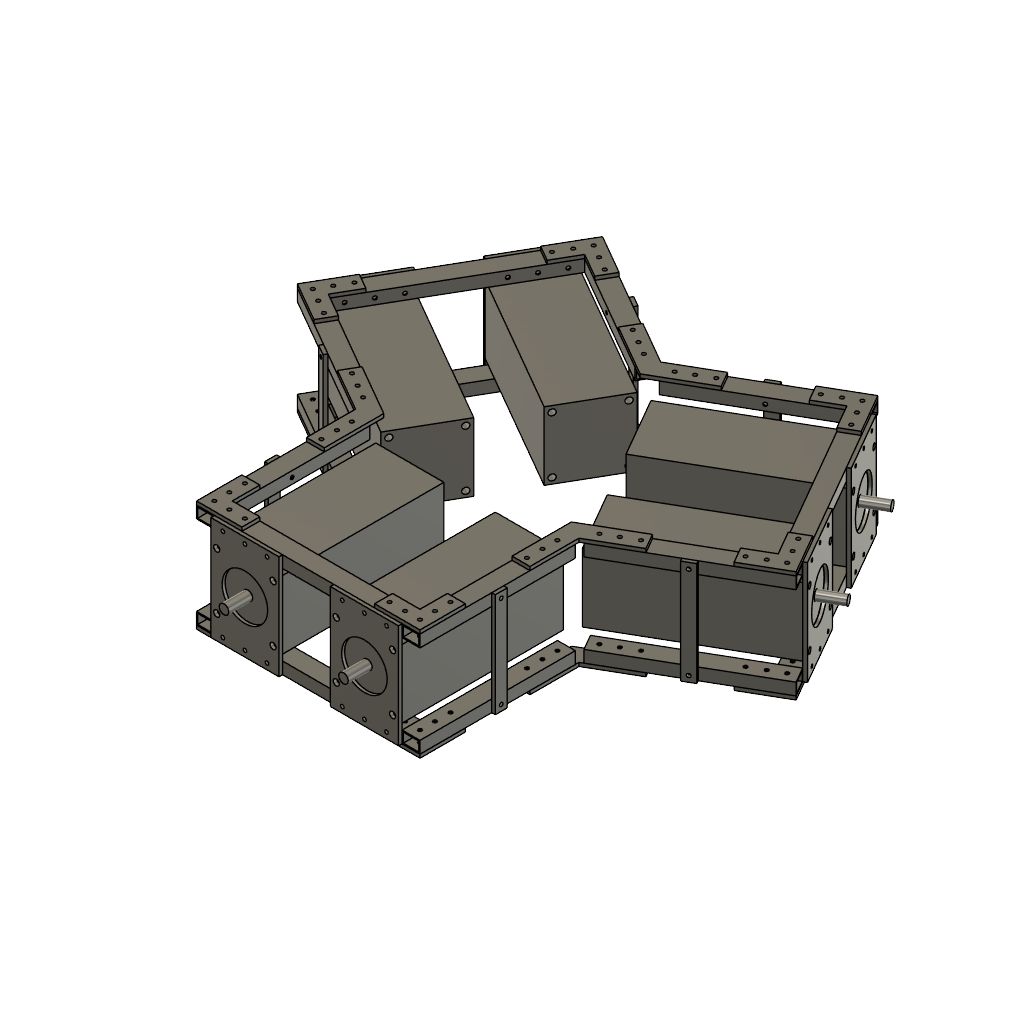
Base (Autodesk Fusion 360 design; units mm, degrees)
Autodesk Fusion 360 part; units mm, degrees
note: some values were not read from the file. Chosen so that the rebuilt part matches the saved one: which bodies a step acts on. Set by a fixed rule: which sketch regions a step uses.
sketch "Sketch1" plane through (0, 0, 0) normal (0, 1, 0) x (1, 0, 0)
  line L0 (0, 0) -> (0, -200)
  line L1 (-50, -200) -> (55.0397, -200)
  line L2 (-21.5, -187) -> (-78.5, -187)
  line L3 (-78.5, -187) -> (-78.5, -52)
  line L4 (-21.5, -187) -> (-21.5, -52)
  line L5 (-78.5, -52) -> (-21.5, -52)
  constraint coincident L0.start origin
  constraint vertical L0
  constraint perpendicular L0 L1
  constraint parallel L1 L2
  constraint perpendicular L2 L3
  constraint perpendicular L2 L4
extrude "Extrude1" add sketch "Sketch1" along normal blind 28.5 makes body 1
move_face "OffsetFaces1" offset 28.5 1 faces at (-59.5, 0, 97) on bodies 1
sketch "Sketch2" plane through (0, 0, 187) normal (0, 0, 1) x (1, 0, 0)
  line L0 (-78.5, -28.5) -> (-21.5, -28.5)
  line L1 (-21.5, -28.5) -> (-21.5, 28.5)
  line L2 (-21.5, 28.5) -> (-78.5, 28.5)
  line L3 (-78.5, 28.5) -> (-78.5, -28.5)
  line L4 (-78.5, 28.5) -> (-21.5, -28.5)
  line L5 (-21.5, 28.5) -> (-78.5, -28.5)
  circle A0 centre (-50, 0) radius 19.05
  constraint coincident L2.end L3.start
  constraint coincident L0.end L1.start
  constraint coincident L1.end L2.start
  constraint coincident L0.start L3.end
  constraint midpoint L5 A0.centre
extrude "Extrude2" add sketch "Sketch2" along normal blind 0.5 contours L4 L5 A0 | L4 L5 A0 | L4 L5 A0 | L4 L5 A0 bodies 1
sketch "Sketch3" plane through (0, 0, 187) normal (0, 0, 1) x (1, 0, 0)
  circle A0 centre (-50, 0) radius 19.05
  line L0 (-78.5, -28.5) -> (-21.5, -28.5)
  line L1 (-21.5, -28.5) -> (-21.5, 28.5)
  line L2 (-21.5, 28.5) -> (-78.5, 28.5)
  line L3 (-78.5, 28.5) -> (-78.5, -28.5)
  line L4 (-26.43, 23.57) -> (-26.43, -23.57)
  line L5 (-26.43, -23.57) -> (-73.57, -23.57)
  line L6 (-73.57, -23.57) -> (-73.57, 23.57)
  line L7 (-73.57, 23.57) -> (-26.43, 23.57)
  circle A1 centre (-73.57, 23.57) radius 2.55
  circle A2 centre (-26.43, 23.57) radius 2.55
  circle A3 centre (-26.43, -23.57) radius 2.55
  circle A4 centre (-73.57, -23.57) radius 2.55
  constraint perpendicular L2 L4
  constraint perpendicular L4 L5
  constraint perpendicular L5 L6
  constraint perpendicular L4 L7
  constraint coincident L6.end L7.start
  constraint coincident L4.start L7.end
  constraint coincident L4.end L5.start
  constraint coincident L5.end L6.start
extrude "Extrude3" cut sketch "Sketch3" against normal blind 135 contours L4 L7 A2 | L4 L7 A2 | L4 L5 A3 | L4 L5 A3 | L6 L7 A1 | L6 L7 A1 | L5 L6 A4 | L5 L6 A4 bodies 1
sketch "Sketch4" plane through (0, 0, 187.5) normal (0, 0, 1) x (1, 0, 0)
  circle A0 centre (-50, 0) radius 19.05
  circle A1 centre (-50, 0) radius 4
  constraint concentric A0 A1
extrude "Extrude4" add sketch "Sketch4" along normal blind 20 contours A1 bodies 1
mirror "Mirror1" about plane through (0, 0, 0) normal (1, 0, 0) of bodies 1 makes body 2
pattern_circular "C-Pattern1" count 3 over 360 about axis through (0, 1.75, 0) along (0, 1, 0) of bodies 1 2 makes body 3 at (113.7545, 28.5, 3.0285) makes body 4 at (-102.7256, 28.5, -106.074) makes body 5 at (54.2545, 28.5, -100.0285) makes body 6 at (-113.7545, 28.5, 3.0285)
sketch "Sketch5" plane through (0, 0, 187) normal (0, 0, 1) x (1, 0, 0)
  circle A0 centre (-73.57, 23.57) radius 2.55
  circle A1 centre (-26.43, 23.57) radius 2.55
  circle A2 centre (-73.57, -23.57) radius 2.55
  circle A3 centre (-26.43, -23.57) radius 2.55
  circle A4 centre (-50, 0) radius 19.05
  line L0 (-78.5, -28.5) -> (-21.5, -28.5)
  line L1 (-21.5, -28.5) -> (-21.5, 28.5)
  line L2 (-21.5, 28.5) -> (-78.5, 28.5)
  line L3 (-78.5, 28.5) -> (-78.5, -28.5)
  line L4 (-83.4322, 43.5) -> (-5, 43.5)
  line L5 (-81, -43.5) -> (-19, -43.5)
  line L6 (-78.5, -28.5) -> (-78.5, -50)
  line L7 (-21.5, -28.5) -> (-21.5, -50)
  line L8 (-21.5, 28.5) -> (-21.5, 50)
  line L9 (-78.5, 28.5) -> (-78.5, 53)
  constraint horizontal L4
  constraint horizontal L5
  constraint coincident L0.start L3.end
  constraint perpendicular L0 L6
  constraint coincident L0.end L1.start
  constraint perpendicular L0 L7
  constraint coincident L1.end L2.start
  constraint perpendicular L2 L8
  constraint coincident L2.end L3.start
  constraint perpendicular L4 L9
extrude "Extrude5" add sketch "Sketch5" along normal blind 3 separate body makes body 7
sketch "Sketch6" plane through (0, 0, 190) normal (0, 0, 1) x (1, 0, 0)
  circle A0 centre (-73.57, 23.57) radius 2.55
  circle A1 centre (-26.43, 23.57) radius 2.55
  circle A2 centre (-26.43, -23.57) radius 2.55
  circle A3 centre (-73.57, -23.57) radius 2.55
  circle A4 centre (-50, 0) radius 19.05
  line L0 (-78.5, 43.5) -> (-78.5, -43.5)
  line L1 (-78.5, -43.5) -> (-21.5, -43.5)
  line L2 (-21.5, -43.5) -> (-21.5, 43.5)
  line L3 (-21.5, 43.5) -> (-78.5, 43.5)
  line L4 (-82, 38.5) -> (-14, 38.5)
  circle A5 centre (-68.5, 38.5) radius 1.5
  circle A6 centre (-31.5, 38.5) radius 1.5
  circle A7 centre (-50, 38.5) radius 1.5
  line L5 (-82.4543, -38.5) -> (-13.292, -38.5) construction
  line L6 (-50, 38.5) -> (-50, -43) construction
  line L7 (-31.5, 38.5) -> (-31.5, -43) construction
  line L8 (-68.5, 38.5) -> (-68.5, -42) construction
  circle A8 centre (-68.5, -38.5) radius 1.5
  circle A9 centre (-50, -38.5) radius 1.5
  circle A10 centre (-31.5, -38.5) radius 1.5
  constraint horizontal L4
  constraint coincident L4 A5.centre
  constraint coincident L4 A6.centre
  constraint coincident L4 A7.centre
  constraint perpendicular L0 L5
  constraint coincident A7.centre L6.start
  constraint perpendicular L1 L6
  constraint coincident A6.centre L7.start
  constraint perpendicular L5 L7
  constraint coincident A5.centre L8.start
  constraint perpendicular L1 L8
  constraint coincident L8 A8.centre
  constraint coincident L5 A8.centre
  constraint coincident L6 A9.centre
  constraint coincident L5 A9.centre
  constraint coincident L7 A10.centre
  constraint coincident L5 A10.centre
extrude "Extrude6" cut sketch "Sketch6" against normal blind 3 contours L4 A5 | L4 A5 | L4 A6 | L4 A6 | L4 A7 | L4 A7 | A8 | A9 | A10 bodies 7
sketch "Sketch7" plane through (0, 0, 187) normal (0, 0, -1) x (-1, 0, 0)
  circle A0 centre (31.5, -38.5) radius 1.5
  circle A1 centre (68.5, 38.5) radius 1.5
  circle A2 centre (50, -38.5) radius 1.5
  circle A3 centre (31.5, 38.5) radius 1.5
  circle A4 centre (50, 38.5) radius 1.5
  circle A5 centre (68.5, -38.5) radius 1.5
  circle A6 centre (73.57, 23.57) radius 2.55
  circle A7 centre (26.43, 23.57) radius 2.55
  circle A8 centre (26.43, -23.57) radius 2.55
  circle A9 centre (73.57, -23.57) radius 2.55
  circle A10 centre (50, 0) radius 19.05
  line L0 (78.5, -43.5) -> (78.5, 43.5)
  line L1 (78.5, 43.5) -> (21.5, 43.5)
  line L2 (21.5, 43.5) -> (21.5, -43.5)
  line L3 (21.5, -43.5) -> (78.5, -43.5)
  line L4 (21.5, 43.5) -> (78.5, 43.5)
  line L5 (78.5, 43.5) -> (78.5, 28.5)
  line L6 (78.5, 28.5) -> (21.5, 28.5)
  line L7 (21.5, 28.5) -> (21.5, 43.5)
  line L8 (18.6686, 33.5) -> (82.3438, 33.5)
  line L9 (-78.5, -28.5) -> (-78.5, 28.5)
  line L10 (-78.5, -7.8499) -> (-78.5, 65.8048)
  line L11 (18.6686, 33.5) -> (-88, 33.5)
  line L12 (21.5, 43.5) -> (-81.618, 43.5)
  constraint horizontal L4
  constraint vertical L5
  constraint horizontal L6
  constraint vertical L7
  constraint coincident L0 L5.end
  constraint coincident L1.end L2.start
  constraint perpendicular L2 L8
  constraint coincident L9 L10.start
  constraint perpendicular L2 L11
  constraint perpendicular L2 L12
extrude "Extrude7" add sketch "Sketch7" along normal blind 15 separate body contours L0 L1 L2 L4 L5 L7 L8 makes body 8
sketch "Sketch8" plane through (-78.5, 0, 0) normal (-1, 0, 0) x (0, 0, 1)
  line L0 (187, 33.5) -> (187, 43.5)
  line L1 (187, 43.5) -> (172, 43.5)
  line L2 (172, 43.5) -> (172, 33.5)
  line L3 (172, 33.5) -> (187, 33.5)
mirror "Mirror2" about plane through (0, 0, 0) normal (1, 0, 0) of bodies 7 makes body 9
pattern_circular "C-Pattern2" count 3 over 360 about axis through (0, 1.75, 0) along (0, 1, 0) of bodies 9 7 makes body 10 at (191.19, 30.8975, -42.8491) makes body 11 at (-132.7035, 30.8975, -144.1509) makes body 12 at (132.7035, -30.8975, -144.1509) makes body 13 at (-191.19, 30.8975, -42.8491)
sketch "Sketch9" plane through (-21.5, 0, 0) normal (1, 0, 0) x (0, 0, -1)
  line L0 (-187, 43.5) -> (-187, 33.5)
  line L1 (-187, 33.5) -> (-172, 33.5)
  line L2 (-172, 33.5) -> (-172, 43.5)
  line L3 (-172, 43.5) -> (-187, 43.5)
sketch "Sketch10" plane through (-21.5, 0, 0) normal (1, 0, 0) x (0, 0, -1)
  line L0 (-187, 43.5) -> (-187, 33.5)
  line L1 (-187, 33.5) -> (-172, 33.5)
  line L2 (-172, 33.5) -> (-172, 43.5)
  line L3 (-172, 43.5) -> (-187, 43.5)
extrude "Extrude8" add sketch "Sketch10" along normal blind 100 separate body makes body 14
combine "Combine1" operation add target body 14 tool bodies 8
sketch "Sketch11" plane through (0, 0, 172) normal (0, 0, -1) x (-1, 0, 0)
  circle A0 centre (31.5, 38.5) radius 1.5
  circle A1 centre (68.5, 38.5) radius 1.5
  circle A2 centre (50, 38.5) radius 1.5
  line L0 (78.5, 43.5) -> (-78.5, 43.5)
  line L1 (-78.5, 43.5) -> (-78.5, 33.5)
  line L2 (-78.5, 33.5) -> (78.5, 33.5)
  line L3 (78.5, 33.5) -> (78.5, 43.5)
  circle A3 centre (-68.5, 38.5) radius 1.5
  circle A4 centre (-50, 38.5) radius 1.5
  circle A5 centre (-31.5, 38.5) radius 1.5
extrude "Extrude9" cut sketch "Sketch11" against normal blind 15 contours A3 | A4 | A5 bodies 14
sketch "Sketch12" plane through (78.5, 0, 0) normal (1, 0, 0) x (0, 0, -1)
  line L0 (-172, 43.5) -> (-187, 43.5)
  line L1 (-187, 43.5) -> (-187, 33.5)
  line L2 (-187, 33.5) -> (-172, 33.5)
  line L3 (-172, 33.5) -> (-172, 43.5)
  line L4 (-187, 43.5) -> (-172, 33.5) construction
  line L5 (-172, 43.5) -> (-187, 33.5) construction
  line L6 (-173, 34.6971) -> (-186, 34.6971)
  line L7 (-186, 34.6971) -> (-186, 42.3029)
  line L8 (-186, 42.3029) -> (-173, 42.3029)
  line L9 (-173, 42.3029) -> (-173, 34.6971)
  line L10 (-173, 34.6971) -> (-186, 42.3029) construction
  line L11 (-186, 34.6971) -> (-173, 42.3029) construction
  point P0 (-179.5, 38.5)
  constraint coincident L0.end L1.start
  constraint coincident L2.end L3.start
  constraint coincident L0.start L3.end
  constraint coincident L1.end L2.start
  constraint horizontal L6
  constraint perpendicular L6 L7
  constraint parallel L6 L8
  constraint parallel L7 L9
  constraint coincident L10 P0
  constraint coincident L11 P0
  constraint midpoint L4 P0
extrude "Extrude10" cut sketch "Sketch12" against normal blind 157 contours L6 L7 L8 L9 bodies 14
sketch "Sketch13" plane through (0, 43.5, 0) normal (0, 1, 0) x (-1, 0, 0)
  line L0 (78.5, 187) -> (-78.5, 187)
  line L1 (-78.5, 187) -> (-78.5, 172)
  line L2 (-78.5, 172) -> (78.5, 172)
  line L3 (78.5, 172) -> (78.5, 187)
  line L4 (55.5, 187) -> (55.5, 172)
  line L5 (73.5, 172) -> (73.5, 187)
  line L6 (60.5, 172) -> (60.5, 187)
  line L7 (78.5, 179.5) -> (42, 179.5) construction
  circle A0 centre (60.5, 179.5) radius 1.5
  circle A1 centre (73.5, 179.5) radius 1.5
  line L8 (-73.5, 170) -> (-73.5, 191.2078)
  line L9 (-60.5, 169.8695) -> (-60.5, 193.8538)
  line L10 (-55.5, 170) -> (-55.5, 195.9898)
  line L11 (-78.5, 179.5) -> (-48.9118, 179.5) construction
  circle A2 centre (-73.5, 179.5) radius 1.5
  circle A3 centre (-60.5, 179.5) radius 1.5
  constraint coincident L0 L4.start
  constraint coincident L2 L4.end
  constraint perpendicular L2 L4
  constraint coincident L2 L5.start
  constraint coincident L0 L5.end
  constraint perpendicular L0 L5
  constraint coincident L2 L6.start
  constraint coincident L0 L6.end
  constraint perpendicular L0 L6
  constraint midpoint L3 L7.start
  constraint perpendicular L3 L7
  constraint midpoint L6 A0.centre
  constraint midpoint L5 A1.centre
  constraint perpendicular L2 L8
  constraint perpendicular L2 L9
  constraint perpendicular L0 L10
  constraint midpoint L1 L11.start
  constraint perpendicular L10 L11
  constraint coincident L8 A2.centre
  constraint coincident L11 A2.centre
  constraint coincident L9 A3.centre
  constraint coincident L11 A3.centre
extrude "Extrude11" cut sketch "Sketch13" against normal blind 10 contours L5 A1 | L5 A1 | L6 A0 | L6 A0 | L9 A3 | L9 A3 | L8 A2 | L8 A2 bodies 14
pattern_circular "C-Pattern3" count 3 over 360 about axis through (0, 1.75, 0) along (0, 1, 0) of bodies 14 makes body 15 at (170.2315, 33.5, -75.1252) makes body 16 at (-150.1761, 33.5, -109.8622)
mirror "Mirror3" about plane through (0, 0, 0) normal (0, 1, 0) of bodies 14 16 15 makes body 17 at (-20.0122, -33.5, 174.0245) makes body 18 at (170.2315, -33.5, -75.1252) makes body 19 at (-150.1761, -33.5, -109.8622)
sketch "Sketch14" plane through (0, 43.5, 0) normal (0, 1, 0) x (-1, 0, 0)
  circle A0 centre (-73.5, 179.5) radius 1.5
  circle A1 centre (73.5, 179.5) radius 1.5
  circle A2 centre (-60.5, 179.5) radius 1.5
  circle A3 centre (60.5, 179.5) radius 1.5
  line L0 (78.5, 187) -> (-78.5, 187)
  line L1 (-78.5, 187) -> (-78.5, 172)
  line L2 (-78.5, 172) -> (78.5, 172)
  line L3 (78.5, 172) -> (78.5, 187)
  line L4 (55.5, 187) -> (55.5, 172)
  circle A4 centre (60.5, 179.5) radius 1.5
  circle A5 centre (73.5, 179.5) radius 1.5
  line L5 (55.5, 187) -> (93.5, 187)
  line L6 (93.5, 187) -> (93.5, 149)
  line L7 (93.5, 149) -> (78.5, 149)
  line L8 (78.5, 149) -> (78.5, 172)
  line L9 (60.5, 179.5) -> (97, 179.5) construction
  line L10 (96, 154) -> (76, 154) construction
  line L11 (97, 167) -> (74, 167) construction
  line L12 (86, 149) -> (86, 187) construction
  circle A6 centre (86, 179.5) radius 1.5
  circle A7 centre (86, 167) radius 1.5
  circle A8 centre (86, 154) radius 1.5
  constraint coincident L4.start L5.start
  constraint perpendicular L3 L5
  constraint vertical L6
  constraint perpendicular L6 L7
  constraint coincident L2.end L3.start
  constraint coincident A3.centre A4.centre
  constraint perpendicular L6 L9
  constraint perpendicular L6 L10
  constraint perpendicular L8 L11
  constraint midpoint L7 L12.start
  constraint coincident L5 L12.end
  constraint perpendicular L5 L12
  constraint coincident L12 A6.centre
  constraint coincident L9 A6.centre
  constraint coincident L12 A7.centre
  constraint coincident L11 A7.centre
  constraint midpoint L10 A8.centre
extrude "Extrude12" add sketch "Sketch14" along normal blind 3 separate body contours L0 L2 L3 L4 L5 | L3 L5 L6 L7 L8 makes body 20
sketch "Sketch15" plane through (0, 43.5, 0) normal (0, -1, 0) x (1, 0, 0)
  circle A0 centre (-86, 179.5) radius 1.5
  circle A1 centre (-86, 154) radius 1.5
  circle A2 centre (-86, 167) radius 1.5
  circle A3 centre (-60.5, 179.5) radius 1.5
  circle A4 centre (-73.5, 179.5) radius 1.5
  line L0 (-55.5, 172) -> (-55.5, 187)
  line L1 (-55.5, 187) -> (-93.5, 187)
  line L2 (-93.5, 187) -> (-93.5, 149)
  line L3 (-93.5, 149) -> (-78.5, 149)
  line L4 (-78.5, 149) -> (-78.5, 172)
  line L5 (-78.5, 172) -> (-55.5, 172)
  line L6 (-21.5, 52) -> (-21.5, 187)
  line L7 (-21.5, 187) -> (-78.5, 187)
  line L8 (-78.5, 187) -> (-78.5, 52)
  line L9 (-78.5, 52) -> (-21.5, 52)
  line L10 (-93.5, 187) -> (-78.5, 187)
  line L11 (-78.5, 187) -> (-78.5, 52)
  line L12 (-78.5, 52) -> (-93.5, 52)
  line L13 (-93.5, 52) -> (-93.5, 187)
  line L14 (-96, 57) -> (-76, 57)
  constraint horizontal L10
  constraint vertical L11
  constraint horizontal L12
  constraint vertical L13
  constraint coincident L8.end L9.start
  constraint coincident L1.end L2.start
  constraint perpendicular L11 L14
extrude "Extrude13" add sketch "Sketch15" along normal blind 10 separate body contours L1 L2 L3 L4 L8 L10 L11 L13 | L3 L8 L11 L13 L14 makes body 21
sketch "Sketch16" plane through (0, 43.5, 0) normal (0, 1, 0) x (-1, 0, 0)
  circle A0 centre (86, 154) radius 1.5
  circle A1 centre (86, 167) radius 1.5
  circle A2 centre (86, 179.5) radius 1.5
  line L0 (93.5, 57) -> (93.5, 187)
  line L1 (93.5, 187) -> (78.5, 187)
  line L2 (78.5, 187) -> (78.5, 57)
  line L3 (78.5, 122) -> (93.5, 122)
  circle A3 centre (86, 90) radius 1.5
  circle A4 centre (86, 77) radius 1.5
  circle A5 centre (86, 64.5) radius 1.5
  line L4 (78.5, 57) -> (93.5, 57)
  constraint midpoint L2 L3.start
  constraint midpoint L0 L3.end
  constraint symmetric A0 L3 A3
  constraint symmetric A1 L3 A4
  constraint symmetric A2 L3 A5
extrude "Extrude14" cut sketch "Sketch16" against normal blind 10 contours A3 | A4 | A5 bodies 21
sketch "Sketch17" plane through (0, 0, 187) normal (0, 0, 1) x (1, 0, 0)
  line L0 (-78.5, 43.5) -> (-93.5, 43.5)
  line L1 (-93.5, 43.5) -> (-93.5, 33.5)
  line L2 (-93.5, 33.5) -> (-78.5, 33.5)
  line L3 (-78.5, 33.5) -> (-78.5, 43.5)
  line L4 (-93.5, 43.5) -> (-78.5, 33.5) construction
  line L5 (-93.5, 33.5) -> (-78.5, 43.5) construction
  line L6 (-79.5, 34.5) -> (-92.5, 34.5)
  line L7 (-92.5, 34.5) -> (-92.5, 42.5)
  line L8 (-92.5, 42.5) -> (-79.5, 42.5)
  line L9 (-79.5, 42.5) -> (-79.5, 34.5)
  line L10 (-79.5, 34.5) -> (-92.5, 42.5) construction
  line L11 (-92.5, 34.5) -> (-79.5, 42.5) construction
  point P0 (-86, 38.5)
  constraint coincident L0.end L1.start
  constraint coincident L2.end L3.start
  constraint coincident L1.end L2.start
  constraint coincident L0.start L3.end
  constraint horizontal L6
  constraint perpendicular L6 L7
  constraint parallel L6 L8
  constraint parallel L7 L9
  constraint coincident L10 P0
  constraint coincident L11 P0
  constraint midpoint L4 P0
extrude "Extrude15" cut sketch "Sketch17" against normal blind 135 contours L6 L7 L8 L9 bodies 21
mirror "Mirror4" about plane through (0, 0, 0) normal (1, 0, 0) of bodies 21 20 makes body 22 at (91.5, 46.5, 167.6667) makes body 23 at (83.7518, 43.5, 131.0107)
mirror "Mirror5" about plane through (0, 0, 0) normal (0, 1, 0) of bodies 21 20 22 23 makes body 24 at (-91.5, -46.5, 167.6667) makes body 25 at (-83.7518, -43.5, 131.0107) makes body 26 at (91.5, -46.5, 167.6667) makes body 27 at (83.7518, -43.5, 131.0107)
pattern_circular "C-Pattern4" count 3 over 360 about axis through (0, 1.75, 0) along (0, 1, 0) of bodies 21 20 22 23 27 25 24 26 makes body 28 at (190.9536, 46.5, -4.592) makes body 29 at (-99.4536, 46.5, -163.0747) makes body 30 at (155.3516, 43.5, 7.0501) makes body 31 at (-71.5702, 33.5, -138.0635) makes body 32 at (99.4536, 46.5, -163.0747) makes body 33 at (-190.9536, 46.5, -4.592) makes body 34 at (71.5702, 43.5, -138.0635) makes body 35 at (-155.3516, 43.5, 7.0501) makes body 36 at (190.9536, -46.5, -4.592) makes body 37 at (-99.4536, -46.5, -163.0747) makes body 38 at (155.3516, -43.5, 7.0501) makes body 39 at (-71.5702, -33.5, -138.0635) makes body 40 at (99.4536, -46.5, -163.0747) makes body 41 at (-190.9536, -46.5, -4.592) makes body 42 at (71.5702, -43.5, -138.0635) makes body 43 at (-155.3516, -43.5, 7.0501)
sketch "Sketch18" plane through (0, 43.5, 0) normal (0, 1, 0) x (-1, 0, 0)
  circle A0 centre (86, 64.5) radius 1.5
  circle A1 centre (86, 77) radius 1.5
  circle A2 centre (86, 90) radius 1.5
  circle A3 centre (86, 167) radius 1.5
  circle A4 centre (86, 179.5) radius 1.5
  circle A5 centre (86, 154) radius 1.5
  line L0 (78.5, 57) -> (93.5, 57)
  line L1 (93.5, 57) -> (93.5, 187)
  line L2 (93.5, 187) -> (78.5, 187)
  line L3 (78.5, 187) -> (78.5, 57)
  circle A6 centre (98.8586, 42.2282) radius 1.5
  circle A7 centre (109.684, 35.9782) radius 1.5
  circle A8 centre (120.9423, 29.4782) radius 1.5
  circle A9 centre (187.6262, -9.0218) radius 1.5
  circle A10 centre (198.4516, -15.2718) radius 1.5
  circle A11 centre (176.3679, -2.5218) radius 1.5
  line L4 (96.1134, 52.4734) -> (88.6134, 39.483)
  line L5 (88.6134, 39.483) -> (201.1968, -25.517)
  line L6 (201.1968, -25.517) -> (208.6968, -12.5266)
  line L7 (208.6968, -12.5266) -> (96.1134, 52.4734)
  line L8 (129.0224, 33.4734) -> (121.5224, 20.483)
  line L9 (93.5, 95) -> (78.5, 95)
  line L10 (106.062, 29.4091) -> (76.1016, 46.7067)
  line L11 (78.5, 65.3387) -> (78.5, 42)
  line L12 (100.3409, 50.0326) -> (92.3394, 54.6523)
  line L13 (93.5, 63.2623) -> (93.5, 52)
  constraint coincident L7 L8.start
  constraint coincident L5 L8.end
  constraint perpendicular L5 L8
  constraint coincident L1 L9.start
  constraint coincident L3 L9.end
  constraint perpendicular L3 L9
  constraint coincident L5 L10.start
  constraint parallel L5 L10
  constraint coincident L3 L11.start
  constraint parallel L3 L11
  constraint coincident L7 L12.start
  constraint parallel L7 L12
  constraint coincident L1 L13.start
  constraint parallel L1 L13
extrude "Extrude16" add sketch "Sketch18" along normal blind 3 separate body contours L0 L1 L3 L9 L11 L13 | L0 L4 L10 L11 L12 L13 | L4 L5 L7 L8 L10 L12 makes body 44
mirror "Mirror6" about plane through (0, 0, 0) normal (0, 1, 0) of bodies 44 makes body 45
pattern_circular "C-Pattern5" count 3 over 360 about axis through (0, 1.75, 0) along (0, 1, 0) of bodies 45 44 makes body 46 at (86.8711, 43.5, 46.2624) makes body 47 at (-3.3711, 43.5, -98.3638) makes body 48 at (86.8711, -43.5, 46.2624) makes body 49 at (-3.3711, -43.5, -98.3638)
sketch "Sketch19" plane through (0, 0, 460) normal (0, 0, 1) x (1, 0, 0)
  circle A0 centre (-31.5, -38.5) radius 1.5
  circle A1 centre (-68.5, 38.5) radius 1.5
  circle A2 centre (-50, -38.5) radius 1.5
  circle A3 centre (-31.5, 38.5) radius 1.5
  circle A4 centre (-50, 38.5) radius 1.5
  circle A5 centre (-68.5, -38.5) radius 1.5
  circle A6 centre (-73.57, 23.57) radius 2.55
  circle A7 centre (-26.43, 23.57) radius 2.55
  circle A8 centre (-26.43, -23.57) radius 2.55
  circle A9 centre (-73.57, -23.57) radius 2.55
  circle A10 centre (-50, 0) radius 19.05
  line L0 (-78.5, 43.5) -> (-78.5, -43.5)
  line L1 (-78.5, -43.5) -> (-21.5, -43.5)
  line L2 (-21.5, -43.5) -> (-21.5, 43.5)
  line L3 (-21.5, 43.5) -> (-78.5, 43.5)
sketch "Sketch20" plane through (0, 43.5, 0) normal (0, 1, 0) x (-1, 0, 0)
  circle A0 centre (-86, 64.5) radius 1.5
  circle A1 centre (-86, 77) radius 1.5
  circle A2 centre (-86, 90) radius 1.5
  circle A3 centre (-86, 167) radius 1.5
  circle A4 centre (-86, 179.5) radius 1.5
  circle A5 centre (-86, 154) radius 1.5
  line L0 (-93.5, 57) -> (-78.5, 57)
  line L1 (-78.5, 57) -> (-78.5, 187)
  line L2 (-78.5, 187) -> (-93.5, 187)
  line L3 (-93.5, 187) -> (-93.5, 57)
sketch "Sketch21" plane through (93.5, 0, 0) normal (1, 0, 0) x (0, 0, -1)
  line L0 (-57, 43.5) -> (-187, 43.5)
  line L1 (-187, 43.5) -> (-187, 33.5)
  line L2 (-187, 33.5) -> (-57, 33.5)
  line L3 (-57, 33.5) -> (-57, 43.5)
  line L4 (-187, -43.5) -> (-57, -43.5)
  line L5 (-57, -43.5) -> (-57, -33.5)
  line L6 (-57, -33.5) -> (-187, -33.5)
  line L7 (-187, -33.5) -> (-187, -43.5)
sketch "Sketch22" plane through (93.5, 0, 0) normal (1, 0, 0) x (0, 0, -1)
  line L0 (-187, -43.5) -> (-57, -43.5)
  line L1 (-57, -43.5) -> (-57, -33.5)
  line L2 (-57, -33.5) -> (-187, -33.5)
  line L3 (-187, -33.5) -> (-187, -43.5)
  line L4 (-57, 43.5) -> (-187, 43.5)
  line L5 (-187, 43.5) -> (-187, 33.5)
  line L6 (-187, 33.5) -> (-57, 33.5)
  line L7 (-57, 33.5) -> (-57, 43.5)
  line L8 (-122, 48.8644) -> (-122, -50) construction
  line L9 (-127, 43.5) -> (-127, -43.5)
  line L10 (-117, 43.5) -> (-117, -43.5)
  constraint perpendicular L2 L8
  constraint coincident L4 L9.start
  constraint coincident L0 L9.end
  constraint perpendicular L0 L9
  constraint coincident L4 L10.start
  constraint coincident L0 L10.end
  constraint perpendicular L0 L10
extrude "Extrude17" add sketch "Sketch22" along normal blind 3 separate body contours L0 L2 L9 L10 | L2 L6 L9 L10 | L4 L6 L9 L10 makes body 50
sketch "Sketch23" plane through (96.5, 0, 0) normal (1, 0, 0) x (0, 0, -1)
  line L0 (-127, 43.5) -> (-127, -43.5)
  line L1 (-127, -43.5) -> (-117, -43.5)
  line L2 (-117, -43.5) -> (-117, 43.5)
  line L3 (-117, 43.5) -> (-127, 43.5)
  line L4 (-127, 43.5) -> (-117, 33.4727) construction
  line L5 (-117, 43.5) -> (-127, 33.5273) construction
  circle A0 centre (-122, 38.4863) radius 1.5
  line L6 (-187, -43.5) -> (-57, -43.5)
  line L7 (-57, -43.5) -> (-57, -33.5)
  line L8 (-57, -33.5) -> (-187, -33.5)
  line L9 (-187, -33.5) -> (-187, -43.5)
  line L10 (-117, -33.5) -> (-127, -43.5) construction
  line L11 (-127, -33.5) -> (-117, -43.5) construction
  circle A1 centre (-122, -38.5) radius 1.5
  constraint coincident L0.start L3.end
  constraint coincident L2 L4.end
  constraint coincident L2.end L3.start
  constraint coincident L0 L5.end
  constraint perpendicular L4 L5
  constraint midpoint L4 A0.centre
  constraint coincident L8 L10.start
  constraint coincident L2 L10.start
  constraint coincident L0.end L1.start
  constraint coincident L0 L11.start
  constraint coincident L8 L11.start
  constraint coincident L1.end L2.start
  constraint midpoint L10 A1.centre
extrude "Extrude18" cut sketch "Sketch23" against normal blind 18 contours A0 | A1 bodies 23 27 50
mirror "Mirror8" about plane through (0, 0, 0) normal (1, 0, 0) of bodies 50 makes body 51
pattern_circular "C-Pattern6" count 3 over 360 about axis through (0, 1.75, 0) along (0, 1, 0) of bodies 51 50 makes body 52 at (55.6282, 12.6118, -140.0815) makes body 53 at (-149.1282, 12.6118, 21.8653) makes body 54 at (150.6282, 12.6118, 24.4634) makes body 55 at (-54.1282, 12.6118, -142.6795)
sketch "Sketch24" plane through (-93.5, 0, 0) normal (-1, 0, 0) x (0, 0, 1)
  line L0 (187, 43.5) -> (57, 43.5)
  line L1 (57, 43.5) -> (57, 33.5)
  line L2 (57, 33.5) -> (187, 33.5)
  line L3 (187, 33.5) -> (187, 43.5)
  circle A0 centre (122, -38.5) radius 1.5
  circle A1 centre (122, 38.4863) radius 1.5
  line L4 (127, -43.5) -> (127, 43.5)
  line L5 (127, 43.5) -> (117, 43.5)
  line L6 (117, 43.5) -> (117, -43.5)
  line L7 (117, -43.5) -> (127, -43.5)
extrude "Extrude19" cut sketch "Sketch24" against normal blind 15 contours A0 | A1 bodies 21 25
sketch "Sketch25" plane through (-46.75, 0, 80.9734) normal (-0.5, 0, 0.866025) x (0.866025, 0, 0.5)
  line L0 (-57, 43.5) -> (-187, 43.5)
  line L1 (-187, 43.5) -> (-187, 33.5)
  line L2 (-187, 33.5) -> (-57, 33.5)
  line L3 (-57, 33.5) -> (-57, 43.5)
  circle A0 centre (-122, -38.5) radius 1.5
  circle A1 centre (-122, 38.4863) radius 1.5
  line L4 (-127, 43.5) -> (-127, -43.5)
  line L5 (-127, -43.5) -> (-117, -43.5)
  line L6 (-117, -43.5) -> (-117, 43.5)
  line L7 (-117, 43.5) -> (-127, 43.5)
extrude "Extrude20" cut sketch "Sketch25" against normal blind 15 contours A0 | A1 bodies 35 43
sketch "Sketch26" plane through (46.75, 0, -80.9734) normal (0.5, 0, -0.866025) x (-0.866025, 0, -0.5)
  line L0 (187, 43.5) -> (57, 43.5)
  line L1 (57, 43.5) -> (57, 33.5)
  line L2 (57, 33.5) -> (187, 33.5)
  line L3 (187, 33.5) -> (187, 43.5)
  circle A0 centre (122, -38.5) radius 1.5
  circle A1 centre (122, 38.4863) radius 1.5
  line L4 (127, -43.5) -> (127, 43.5)
  line L5 (127, 43.5) -> (117, 43.5)
  line L6 (117, 43.5) -> (117, -43.5)
  line L7 (117, -43.5) -> (127, -43.5)
extrude "Extrude21" cut sketch "Sketch26" against normal blind 15 contours A0 | A1 bodies 31 39
sketch "Sketch27" plane through (-46.75, 0, -80.9734) normal (-0.5, 0, -0.866025) x (-0.866025, 0, 0.5)
  line L0 (-187, -43.5) -> (-57, -43.5)
  line L1 (-57, -43.5) -> (-57, -33.5)
  line L2 (-57, -33.5) -> (-187, -33.5)
  line L3 (-187, -33.5) -> (-187, -43.5)
  circle A0 centre (-122, -38.5) radius 1.5
  circle A1 centre (-122, 38.4863) radius 1.5
  line L4 (-127, 43.5) -> (-127, -43.5)
  line L5 (-127, -43.5) -> (-117, -43.5)
  line L6 (-117, -43.5) -> (-117, 43.5)
  line L7 (-117, 43.5) -> (-127, 43.5)
extrude "Extrude22" cut sketch "Sketch27" against normal blind 15 contours A0 | A1 bodies 34 42
sketch "Sketch28" plane through (46.75, 0, 80.9734) normal (0.5, 0, 0.866025) x (0.866025, 0, -0.5)
  line L0 (187, 43.5) -> (57, 43.5)
  line L1 (57, 43.5) -> (57, 33.5)
  line L2 (57, 33.5) -> (187, 33.5)
  line L3 (187, 33.5) -> (187, 43.5)
  circle A0 centre (122, -38.5) radius 1.5
  circle A1 centre (122, 38.4863) radius 1.5
  line L4 (127, -43.5) -> (127, 43.5)
  line L5 (127, 43.5) -> (117, 43.5)
  line L6 (117, 43.5) -> (117, -43.5)
  line L7 (117, -43.5) -> (127, -43.5)
extrude "Extrude23" cut sketch "Sketch28" against normal blind 15 contours A0 | A1 bodies 30 38
copy_body "CopyPasteBodies6" bodies 50 makes body 56
move_body "Move13" bodies 56 to x (0, 1, 0) y (-1, 0, 0) z (0, 0, 1) at (50, -137, 200)
copy_body "CopyPasteBodies10" bodies 56 makes body 57
move_body "Move19" bodies 57 to x (1, 0, 0) y (0, 1, 0) z (0, 0, 1) at (0, 0, 15)
copy_body "CopyPasteBodies11" bodies 57 makes body 58
move_body "Move20" bodies 58 to x (1, 0, 0) y (0, 1, 0) z (0, 0, 1) at (0, 0, 15)
copy_body "CopyPasteBodies12" bodies 46 makes body 59
move_body "Move21" bodies 59 to x (1, 0, 0) y (0, 1, 0) z (0, 0, 1) at (240, -110, 0)
copy_body "CopyPasteBodies13" bodies 59 makes body 60
move_body "Move22" bodies 60 to x (1, 0, 0) y (0, 1, 0) z (0, 0, 1) at (20, 0, 10)
move_body "Move23" bodies 59 60 to x (0.5, 0, 0.866025) y (0, 1, 0) z (-0.866025, 0, 0.5) at (176.9888, 0, -265.5876)
hidden bodies 56 57 58 59 60
